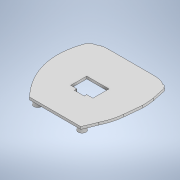
# Autodesk Inventor part: 장갑_위_찐
Saved by Autodesk Inventor 2022 (Build 260153000, 153)
## iProperties
Created: 2023-11-21
Part Number: 장갑_위_찐
Material: 일반
Document SubType Name: Modeling
Designer: USER
Density: 1 g/cm^3
Appearance: 기본값
Author: USER
Autodesk Inventor part; units mm, degrees
ref_plane "YZ Plane" through (0, 0, 0) normal (1, 0, 0) x (0, 1, 0)
ref_plane "XY Plane" through (0, 0, 0) normal (0, 0, 1) x (1, 0, 0)
ref_plane "작업 평면16" through (0, -21, 0) normal (0, 1, 0) x (-1, 0, 0)
sketch "스케치46" plane through (0, -21, 0) normal (0, 1, 0) x (-1, 0, 0)
  spline S0 degree 3 poles (191.4874, -85.0161) (195.7231, -69.6387) (195.5194, -54.7481) (188.0983, -31.7262) (183.731, -23.2823) (177.7743, -15.0127) knots 0.143885 0.143885 0.143885 0.143885 0.581431 0.581431 0.843231 0.843231 0.843231 0.843231
  spline S1 degree 3 poles (189.2538, -92.0465) (190.1005, -89.6919) (190.845, -87.3484) (191.4874, -85.0161) knots 0.077523 0.077523 0.077523 0.077523 0.143885 0.143885 0.143885 0.143885
  arc A0 (183.4058, -96.885) -> (189.2538, -92.0465) centre (181.526, -88.6596) ccw
  spline S2 degree 3 poles (177.1168, -99.3875) (178.1345, -99.0781) (179.1243, -98.6874) (180.7924, -97.822) (181.4844, -97.3903) (182.1335, -96.8989) knots -0.627135 -0.627135 -0.627135 -0.627135 -0.308629 -0.308629 -0.063964 -0.063964 -0.063964 -0.063964
  ellipse E0 centre (180.8973, -97.418) end of major axis (175.52, -97.6575) minor radius 0.4767 (183.4058, -96.885) -> (182.1335, -96.8989) ccw
  spline S3 degree 3 poles (169.3014, -100.3265) (170.1206, -100.3155) (170.9637, -100.2934) (173.5928, -100.1416) (175.3872, -99.9134) (177.1168, -99.3875) knots -0.790866 -0.790866 -0.790866 -0.790866 -0.54231 -0.54231 0 0 0 0
  ellipse E1 centre (154.0427, -99.7705) end of major axis (172.6036, -100.1468) minor radius 0.4335 (166.2054, -100.3445) -> (169.3014, -100.3265) ccw
  line L0 (117.5358, -100.3445) -> (166.2054, -100.3445)
  spline S4 degree 3 poles (177.7743, -15.0127) (174.6367, -10.6567) (171.058, -6.3491) (167.0384, -2.0899) knots 0.843231 0.843231 0.843231 0.843231 0.981134 0.981134 0.981134 0.981134
  line L1 (167.0384, -2.0899) -> (104.9322, -2.0899)
  spline S5 degree 3 poles (104.9322, -2.0899) (102.452, -7.1506) (100.3104, -12.2796) (98.5075, -17.477) knots 0.836147 0.836147 0.836147 0.836147 1 1 1 1
  spline S6 degree 3 poles (98.5075, -17.477) (97.9178, -18.6748) (97.3597, -19.8935) (96.0924, -22.888) (95.4222, -24.6714) (94.4856, -27.5216) (94.1741, -28.5502) (93.7016, -30.2529) (93.5277, -30.9181) (93.2089, -32.2157) (93.0634, -32.8461) (92.745, -34.3177) (92.5794, -35.1581) (92.103, -37.8278) (91.8501, -39.6604) (91.6665, -41.4919) knots -2.526004 -2.526004 -2.526004 -2.526004 -2.120534 -2.120534 -1.544298 -1.544298 -1.220936 -1.220936 -1.014307 -1.014307 -0.819565 -0.819565 -0.560995 -0.560995 0 0 0 0
  line L2 (91.6665, -41.4919) -> (89.5894, -62.2122)
  spline S7 degree 3 poles (89.5894, -62.2122) (89.5894, -63.3351) (89.6133, -64.4561) (89.6986, -66.503) (89.7523, -67.4237) (89.8984, -69.389) (89.9946, -70.4286) (90.2978, -73.1917) (90.5351, -74.9036) (90.8157, -76.6062) knots -1.44821 -1.44821 -1.44821 -1.44821 -1.11115 -1.11115 -0.834292 -0.834292 -0.520567 -0.520567 0 0 0 0
  line L3 (90.8157, -76.6062) -> (94.465, -93.7314)
  arc A1 (94.465, -93.7314) -> (95.652, -93.9327) centre (165.2915, 320.1429) ccw
  ellipse E2 centre (105.5879, -87.8445) end of major axis (105.5879, -100.3445) minor radius 11.3766 (95.652, -93.9327) -> (96.6978, -95.6442) ccw
  arc A2 (96.6978, -95.6442) -> (98.3748, -96.4646) centre (98.7561, -93.561) ccw
  ellipse E3 centre (102.6075, -95.7007) end of major axis (109.3466, -95.2724) minor radius 0.6378 (98.3748, -96.4646) -> (99.6471, -96.4613) ccw
  spline S8 degree 3 poles (99.6471, -96.4613) (100.4112, -97.0879) (101.245, -97.6223) (103.148, -98.5885) (104.2178, -98.9855) (107.048, -99.7682) (109.0052, -100.0586) (111.2899, -100.1922) knots -1.504226 -1.504226 -1.504226 -1.504226 -1.123667 -1.123667 -0.686597 -0.686597 0 0 0 0
  spline S9 degree 3 poles (111.2899, -100.1922) (113.3488, -100.3126) (115.5027, -100.3445) (117.5358, -100.3445) knots -0.609915 -0.609915 -0.609915 -0.609915 0 0 0 0
  line L4 (117.5358, -100.3445) -> (166.2054, -100.3445)
  ellipse E4 centre (154.0427, -99.7705) end of major axis (172.6036, -100.1468) minor radius 0.4335 (166.2054, -100.3445) -> (169.3014, -100.3265) ccw
  spline S10 degree 3 poles (169.3014, -100.3265) (170.1206, -100.3155) (170.9637, -100.2934) (173.5928, -100.1416) (175.3872, -99.9134) (177.1168, -99.3875) knots -0.790866 -0.790866 -0.790866 -0.790866 -0.54231 -0.54231 0 0 0 0
  spline S11 degree 3 poles (177.1168, -99.3875) (178.1345, -99.0781) (179.1243, -98.6874) (180.7924, -97.822) (181.4844, -97.3903) (182.1335, -96.8989) knots -0.627135 -0.627135 -0.627135 -0.627135 -0.308629 -0.308629 -0.063964 -0.063964 -0.063964 -0.063964
  ellipse E5 centre (180.8973, -97.418) end of major axis (175.52, -97.6575) minor radius 0.4767 (183.4058, -96.885) -> (182.1335, -96.8989) ccw
  arc A3 (183.4058, -96.885) -> (189.2538, -92.0465) centre (181.526, -88.6596) ccw
  spline S12 degree 3 poles (189.2538, -92.0465) (190.1005, -89.6919) (190.845, -87.3484) (191.4874, -85.0161) knots 0.077523 0.077523 0.077523 0.077523 0.143885 0.143885 0.143885 0.143885
  spline S13 degree 3 poles (191.4874, -85.0161) (195.7231, -69.6387) (195.5194, -54.7481) (188.0983, -31.7262) (183.731, -23.2823) (177.7743, -15.0127) knots 0.143885 0.143885 0.143885 0.143885 0.581431 0.581431 0.843231 0.843231 0.843231 0.843231
  spline S14 degree 3 poles (189.5592, -84.485) (189.4545, -84.8653) (189.2663, -85.5314) (189.0415, -86.2939) (188.8686, -86.8664) (188.7513, -87.2483) (188.602, -87.7261) (188.4805, -88.1086) (188.326, -88.587) (188.2003, -88.9701) (188.0405, -89.4492) (187.9106, -89.8328) (187.7456, -90.3127) (187.5779, -90.7929) (187.441, -91.1774) (187.3718, -91.3698) knots 0.077523 0.077523 0.077523 0.077523 0.088583 0.096878 0.099644 0.105174 0.107939 0.113469 0.116234 0.121764 0.124529 0.130059 0.132824 0.138354 0.143885 0.143885 0.143885 0.143885
  arc A4 (180.8973, -95.3262) -> (187.3718, -91.3698) centre (181.2393, -88.61) ccw
  spline S15 degree 3 poles (180.8973, -95.3262) (180.6943, -95.4789) (180.3216, -95.7405) (179.8747, -96.018) (179.5233, -96.221) (179.2849, -96.3513) (178.9819, -96.5081) (178.7361, -96.6283) (178.4248, -96.7723) (178.1725, -96.8825) (177.8532, -97.0141) (177.5947, -97.1146) (177.268, -97.2343) (176.9377, -97.3481) (176.6698, -97.433) (176.535, -97.474) knots -0.622898 -0.622898 -0.622898 -0.622898 -0.533273 -0.462877 -0.439411 -0.39248 -0.369015 -0.322084 -0.298619 -0.251688 -0.228222 -0.181292 -0.157826 -0.110895 -0.063964 -0.063964 -0.063964 -0.063964
  line L5 (176.535, -97.474) -> (111.4067, -98.1956)
  spline S16 degree 3 poles (111.4067, -98.1956) (111.0082, -98.1723) (110.2355, -98.1159) (109.3273, -98.0206) (108.4602, -97.9064) (107.7985, -97.7999) (107.0879, -97.6629) (106.6323, -97.562) (106.2272, -97.4625) (106.0103, -97.4058) (105.7968, -97.3472) (105.6552, -97.307) (105.3736, -97.224) (105.0254, -97.1142) (104.5121, -96.935) (104.1099, -96.7784) (103.7148, -96.6109) (103.455, -96.4936) (103.1348, -96.3398) (102.8824, -96.2109) (102.573, -96.043) (102.3302, -95.9032) (101.9734, -95.685) (101.5109, -95.3793) (101.1273, -95.0886) (100.9153, -94.9147) knots 0 0 0 0 0.125352 0.250704 0.31338 0.438733 0.501409 0.595423 0.626761 0.673768 0.689437 0.720775 0.736444 0.814789 0.877465 0.971479 1.002817 1.065493 1.096832 1.159508 1.190846 1.253522 1.28486 1.378874 1.504226 1.504226 1.504226 1.504226
  arc A5 (96.293, -91.0501) -> (100.9153, -94.9147) centre (102.2083, -88.6716) ccw
  arc A6 (92.3068, -61.3872) -> (96.293, -91.0501) centre (227.7562, -58.2846) ccw
  arc A7 (107.3313, -4.0899) -> (92.3068, -61.3872) centre (218.4178, -63.8374) ccw
  line L6 (107.3313, -4.0899) -> (166.1723, -4.0899)
  spline S17 degree 3 poles (166.1723, -4.0899) (166.7932, -4.7558) (167.8603, -5.9228) (169.041, -7.2601) (169.91, -8.2645) (170.4809, -8.9348) (171.1843, -9.7736) (171.7386, -10.4454) (172.4212, -11.286) (172.959, -11.9593) (173.6208, -12.8017) (174.142, -13.4764) (174.7831, -14.3207) (175.4139, -15.1658) (175.9075, -15.8429) (176.1515, -16.1817) knots 0.843231 0.843231 0.843231 0.843231 0.865071 0.881452 0.886912 0.897832 0.903292 0.914212 0.919672 0.930592 0.936052 0.946972 0.952432 0.963352 0.974272 0.974272 0.974272 0.974272
  spline S18 degree 3 poles (176.1515, -16.1817) (177.4538, -17.9897) (179.9013, -21.6192) (182.5692, -26.1898) (184.9446, -30.7857) (186.6116, -34.4828) (188.4049, -39.1304) (189.6076, -42.8697) (190.8225, -47.5717) (191.5638, -51.3563) (192.2029, -56.1175) (192.4844, -59.9515) (192.5489, -64.7775) (192.3706, -68.6656) (191.8595, -73.5618) (191.0598, -78.4947) (190.1111, -82.4814) (189.5592, -84.485) knots 0.143885 0.143885 0.143885 0.143885 0.202163 0.260442 0.289582 0.347861 0.377 0.435279 0.464418 0.522697 0.551837 0.610116 0.639255 0.697534 0.726673 0.784952 0.843231 0.843231 0.843231 0.843231
  circle A8 centre (157.0041, -93.6029) radius 2.75
  circle A9 centre (157.0041, -93.6029) radius 4.75
  line L7 (176.535, -97.474) -> (111.4067, -98.1956)
  circle A10 centre (164.2713, -9.3093) radius 2.75
  circle A11 centre (164.2713, -9.3093) radius 4.75
  circle A12 centre (110.4218, -9.3093) radius 2.75
  circle A13 centre (110.4218, -9.3093) radius 4.75
  line L8 (154.2569, -58.8887) -> (127.2569, -58.8887)
  line L9 (127.2569, -58.8887) -> (127.2569, -39.3887)
  line L10 (154.2569, -39.3887) -> (154.2569, -58.8887)
  line L11 (146.7569, -39.3887) -> (146.7569, -36.3887)
  line L12 (146.7569, -36.3887) -> (134.7569, -36.3887)
  line L13 (134.7569, -36.3887) -> (134.7569, -39.3887)
  line L14 (127.2569, -39.3887) -> (134.7569, -39.3887)
  line L15 (146.7569, -39.3887) -> (154.2569, -39.3887)
  line L16 (121.2569, -62.8887) -> (160.2569, -62.8887)
  line L17 (160.2569, -62.8887) -> (160.2569, -34.8887)
  line L18 (160.2569, -34.8887) -> (121.2569, -34.8887)
  line L19 (121.2569, -34.8887) -> (121.2569, -62.8887)
  line L20 (162.2569, -64.8887) -> (119.2569, -64.8887)
  line L21 (119.2569, -64.8887) -> (119.2569, -32.8887)
  line L22 (119.2569, -32.8887) -> (162.2569, -32.8887)
  line L23 (162.2569, -32.8887) -> (162.2569, -64.8887)
  line L24 (136.7569, -62.8887) -> (136.7569, -64.8887)
  line L25 (144.7569, -62.8887) -> (144.7569, -64.8887)
  line L26 (140.7569, -58.8887) -> (140.7569, -78.8674)
  point P0 (0, 0)
  point P1 (135.3739, -0.3445)
  point P2 (177.7743, -15.0127)
  point P3 (159.4693, -97.6631)
  point P4 (154.6295, -97.7167)
  dimension "d272" = 5.5
  dimension "d273" = 2
  dimension "d274" = 5.5
  dimension "d275" = 2
  dimension "d276" = 5.5
  dimension "d277" = 2
  dimension "d284" = 27
  dimension "d285" = 19.5
  dimension "d286" = 12
  dimension "d287" = 7.5
  dimension "d288" = 3
  dimension "d291" = 3
  dimension "d292" = 39
  dimension "d293" = 28
  dimension "d294" = 6
  dimension "d295" = 4
  dimension "d296" = 2
  dimension "d297" = 4
  dimension "d298" = 4
  constraints: 54 end point, 16 point on circle, 14 centre point, 8 perpendicular, 7 parallel, 4 point on line, 3 vertical, 2 horizontal, 1 midpoint, 77 other
  measures "d272" diameter of A8
  measures "d273" radial gap between concentric circles of A8 A9
  measures "d274" diameter of A10
  measures "d275" radial gap between concentric circles of A10 A11
  measures "d276" diameter of A12
  measures "d277" radial gap between concentric circles of A12 A13
  measures "d284" distance of L8.start L8.end
  measures "d285" distance of L8.end L9.end
  measures "d286" distance of L11.end L12.end
  measures "d287" distance between parallel lines of L11 L10
  measures "d288" distance of L12.end L13.end
  measures "d291" distance between parallel lines of L15 L12
  measures "d292" distance of L16.start L16.end
  measures "d293" distance of L16.end L17.end
  measures "d294" distance between parallel lines of L17 L10
  measures "d295" distance between parallel lines of L16 L8
  measures "d296" distance between parallel lines of L16 L20
  measures "d297" distance between parallel lines of L24 L26
  measures "d298" distance between parallel lines of L25 L26
extrude "돌출51" add sketch "스케치46" along normal blind 3 contours S1 A0 E0 S2 S3 E1 L0 S9 S8 E3 A2 E2 A1 L3 S7 L2 S6 S5 L1 S4 S0 | S14 A4 S15 L5 A9 S16 A5 A6 A7 L6 S17 S18 | A9 L5 | L5 A9 | A8 | A10 | A11 | A12 | A13 | L16 L19 L18 L17 | L16 L25 L20 L26 | L26 L20 L24 L16 | L8 L9 L14 L13 L12 L11 L15 L10 | L24 L20 L21 L22 L23 L25 L16 L17 L18 L19
extrude "돌출53" add sketch "스케치46" against normal blind 7 contours A9 L5 | L5 A9 | A11 | A13
extrude "돌출54" cut sketch "스케치46" along normal blind 7 contours L8 L9 L14 L13 L12 L11 L15 L10
extrude "돌출55" add sketch "스케치46" against normal blind 3 contours L24 L20 L21 L22 L23 L25 L16 L17 L18 L19
